Autodesk Inventor part; units mm, degrees
(part 2 of 2)
  spline S29 degree 3 poles (44.5449, -33.6903) (44.3882, -33.8514) (44.153, -34.0929) (43.8555, -34.4298) (43.6383, -34.6876) (43.4284, -34.9513) (43.2262, -35.221) (43.0325, -35.497) (42.8484, -35.7793) (42.6754, -36.0687) (42.5143, -36.3649) (42.3963, -36.6199) (42.3064, -36.8258) (42.2261, -36.9743) (42.1307, -37.1135) (42.0181, -37.2395) (41.9088, -37.3284) (41.8141, -37.3893) (41.7375, -37.4246) (41.6598, -37.4575) (41.5776, -37.4771) (41.4949, -37.4937) (41.4105, -37.496) (41.326, -37.4951) (41.2151, -37.4757) (41.0784, -37.444) (40.9405, -37.4173) (40.8313, -37.39) (40.7538, -37.3564) (40.6776, -37.32) (40.6088, -37.2711) (40.5417, -37.2199) (40.484, -37.1582) (40.4284, -37.0947) (40.3668, -37.0006) (40.303, -36.875) (40.2514, -36.714) (40.2209, -36.548) (40.2079, -36.3798) (40.2096, -36.1551) (40.2054, -35.8742) (40.1788, -35.538) (40.1384, -35.2033) (40.0851, -34.8705) (40.0204, -34.5396) (39.9454, -34.211) (39.8609, -33.8847) (39.7673, -33.5608) (39.6325, -33.1321) (39.5159, -32.8158) (39.4382, -32.6049) knots -1.0784 -1.0784 -1.0784 -1.0784 -1.010995 -0.977291 -0.943586 -0.909882 -0.876178 -0.842474 -0.80877 -0.775067 -0.741365 -0.707665 -0.690816 -0.67397 -0.657123 -0.640284 -0.623449 -0.615023 -0.606598 -0.598176 -0.589749 -0.581327 -0.572901 -0.564477 -0.556053 -0.5392 -0.522347 -0.513923 -0.505499 -0.497074 -0.488651 -0.480225 -0.471802 -0.463377 -0.454951 -0.438116 -0.421277 -0.40443 -0.387584 -0.370735 -0.337035 -0.303333 -0.26963 -0.235926 -0.202222 -0.168518 -0.134814 -0.101109 -0.067405 0 0 0 0 construction
  arc A24 (39.4382, -32.6049) -> (37.971, -32.4507) centre (35.3606, -64.344) ccw construction
  spline S30 degree 3 poles (37.971, -32.4507) (37.8511, -32.6408) (37.6713, -32.9259) (37.4503, -33.3173) (37.2915, -33.6146) (37.141, -33.9162) (36.9993, -34.2221) (36.8672, -34.5323) (36.7458, -34.8467) (36.6368, -35.1657) (36.5408, -35.489) (36.4784, -35.7629) (36.4333, -35.983) (36.3856, -36.1449) (36.3212, -36.3009) (36.2373, -36.4477) (36.1488, -36.5573) (36.0689, -36.6365) (36.0013, -36.687) (35.9321, -36.7354) (35.8558, -36.7716) (35.7783, -36.8051) (35.6962, -36.8249) (35.6135, -36.8416) (35.5009, -36.8456) (35.3606, -36.843) (35.2202, -36.8456) (35.1077, -36.8416) (35.0249, -36.8249) (34.9428, -36.8051) (34.8653, -36.7716) (34.789, -36.7354) (34.7198, -36.687) (34.6523, -36.6365) (34.5723, -36.5573) (34.4839, -36.4477) (34.4, -36.3009) (34.3355, -36.1449) (34.2879, -35.983) (34.2428, -35.7629) (34.1803, -35.489) (34.0844, -35.1657) (33.9753, -34.8467) (33.8539, -34.5323) (33.7219, -34.2221) (33.5802, -33.9162) (33.4297, -33.6146) (33.2709, -33.3173) (33.0498, -32.9259) (32.87, -32.6408) (32.7502, -32.4507) knots -1.0784 -1.0784 -1.0784 -1.0784 -1.010995 -0.977291 -0.943586 -0.909882 -0.876178 -0.842474 -0.80877 -0.775067 -0.741365 -0.707665 -0.690816 -0.67397 -0.657123 -0.640284 -0.623449 -0.615023 -0.606598 -0.598176 -0.589749 -0.581327 -0.572901 -0.564477 -0.556053 -0.5392 -0.522347 -0.513923 -0.505499 -0.497074 -0.488651 -0.480225 -0.471802 -0.463377 -0.454951 -0.438116 -0.421277 -0.40443 -0.387584 -0.370735 -0.337035 -0.303333 -0.26963 -0.235926 -0.202222 -0.168518 -0.134814 -0.101109 -0.067405 0 0 0 0 construction
  arc A25 (32.7502, -32.4507) -> (31.2829, -32.6049) centre (35.3606, -64.344) ccw construction
  spline S31 degree 3 poles (31.2829, -32.6049) (31.2052, -32.8158) (31.0887, -33.1321) (30.9538, -33.5608) (30.8603, -33.8847) (30.7758, -34.211) (30.7008, -34.5396) (30.6361, -34.8705) (30.5827, -35.2033) (30.5424, -35.538) (30.5157, -35.8742) (30.5116, -36.1551) (30.5133, -36.3798) (30.5003, -36.548) (30.4697, -36.714) (30.4181, -36.875) (30.3544, -37.0006) (30.2927, -37.0947) (30.2371, -37.1582) (30.1795, -37.2199) (30.1124, -37.2711) (30.0435, -37.32) (29.9673, -37.3564) (29.8899, -37.39) (29.7806, -37.4173) (29.6428, -37.444) (29.506, -37.4757) (29.3951, -37.4951) (29.3107, -37.496) (29.2263, -37.4937) (29.1435, -37.4771) (29.0614, -37.4575) (28.9836, -37.4246) (28.907, -37.3893) (28.8124, -37.3284) (28.7031, -37.2395) (28.5905, -37.1135) (28.495, -36.9743) (28.4147, -36.8258) (28.3249, -36.6199) (28.2068, -36.3649) (28.0458, -36.0687) (27.8728, -35.7793) (27.6886, -35.497) (27.495, -35.221) (27.2928, -34.9513) (27.0829, -34.6876) (26.8657, -34.4298) (26.5681, -34.0929) (26.333, -33.8514) (26.1762, -33.6903) knots -1.0784 -1.0784 -1.0784 -1.0784 -1.010995 -0.977291 -0.943586 -0.909882 -0.876178 -0.842474 -0.80877 -0.775067 -0.741365 -0.707665 -0.690816 -0.67397 -0.657123 -0.640284 -0.623449 -0.615023 -0.606598 -0.598176 -0.589749 -0.581327 -0.572901 -0.564477 -0.556053 -0.5392 -0.522347 -0.513923 -0.505499 -0.497074 -0.488651 -0.480225 -0.471802 -0.463377 -0.454951 -0.438116 -0.421277 -0.40443 -0.387584 -0.370735 -0.337035 -0.303333 -0.26963 -0.235926 -0.202222 -0.168518 -0.134814 -0.101109 -0.067405 0 0 0 0 construction
  arc A26 (26.1762, -33.6903) -> (24.7731, -34.1463) centre (35.3606, -64.344) ccw construction
  spline S32 degree 3 poles (24.7731, -34.1463) (24.7409, -34.3687) (24.6927, -34.7023) (24.6499, -35.1497) (24.6258, -35.4859) (24.611, -35.8227) (24.6059, -36.1598) (24.6114, -36.4968) (24.6284, -36.8335) (24.6586, -37.1692) (24.7024, -37.5036) (24.7567, -37.7792) (24.8051, -37.9987) (24.8274, -38.1659) (24.832, -38.3347) (24.815, -38.5028) (24.7788, -38.639) (24.738, -38.7439) (24.6968, -38.8175) (24.6533, -38.8898) (24.5983, -38.9539) (24.5411, -39.016) (24.4742, -39.0675) (24.4054, -39.1164) (24.3042, -39.1658) (24.1749, -39.2206) (24.0477, -39.28) (23.9433, -39.3221) (23.8609, -39.3405) (23.7778, -39.3558) (23.6934, -39.3568) (23.609, -39.3548) (23.5261, -39.3387) (23.4438, -39.3201) (23.3386, -39.2802) (23.2132, -39.216) (23.0769, -39.1161) (22.9546, -38.9998) (22.8452, -38.8713) (22.7144, -38.6885) (22.546, -38.4637) (22.3268, -38.2074) (22.0975, -37.9603) (21.8587, -37.7224) (21.6119, -37.4928) (21.358, -37.271) (21.0978, -37.0567) (20.8318, -36.8497) (20.4707, -36.582) (20.1905, -36.3946) (20.0037, -36.2697) knots -1.0784 -1.0784 -1.0784 -1.0784 -1.010995 -0.977291 -0.943586 -0.909882 -0.876178 -0.842474 -0.80877 -0.775067 -0.741365 -0.707665 -0.690816 -0.67397 -0.657123 -0.640284 -0.623449 -0.615023 -0.606598 -0.598176 -0.589749 -0.581327 -0.572901 -0.564477 -0.556053 -0.5392 -0.522347 -0.513923 -0.505499 -0.497074 -0.488651 -0.480225 -0.471802 -0.463377 -0.454951 -0.438116 -0.421277 -0.40443 -0.387584 -0.370735 -0.337035 -0.303333 -0.26963 -0.235926 -0.202222 -0.168518 -0.134814 -0.101109 -0.067405 0 0 0 0 construction
  arc A27 (20.0037, -36.2697) -> (18.726, -37.0074) centre (35.3606, -64.344) ccw construction
  spline S33 degree 3 poles (18.726, -37.0074) (18.7408, -37.2317) (18.7629, -37.568) (18.8141, -38.0146) (18.8604, -38.3484) (18.916, -38.6809) (18.9811, -39.0117) (19.0566, -39.3402) (19.1432, -39.666) (19.2425, -39.9882) (19.3549, -40.3061) (19.4653, -40.5644) (19.5582, -40.769) (19.6148, -40.928) (19.6544, -41.092) (19.6728, -41.2601) (19.6656, -41.4008) (19.6476, -41.5119) (19.6226, -41.5924) (19.595, -41.6722) (19.5546, -41.7463) (19.5115, -41.819) (19.4568, -41.8833) (19.3997, -41.9454) (19.3109, -42.0148) (19.1959, -42.0952) (19.0838, -42.1798) (18.9904, -42.2427) (18.9137, -42.2778) (18.8356, -42.3101) (18.7532, -42.3285) (18.6703, -42.3441) (18.5858, -42.3457) (18.5015, -42.3445) (18.3903, -42.3274) (18.2542, -42.2907) (18.1001, -42.2213) (17.9563, -42.133) (17.8226, -42.03) (17.6567, -41.8784) (17.4452, -41.6935) (17.1775, -41.4884) (16.9018, -41.2944) (16.6188, -41.1114) (16.3296, -40.9381) (16.0352, -40.7739) (15.7361, -40.6184) (15.4329, -40.4712) (15.0241, -40.2845) (14.711, -40.1594) (14.5023, -40.0761) knots -1.0784 -1.0784 -1.0784 -1.0784 -1.010995 -0.977291 -0.943586 -0.909882 -0.876178 -0.842474 -0.80877 -0.775067 -0.741365 -0.707665 -0.690816 -0.67397 -0.657123 -0.640284 -0.623449 -0.615023 -0.606598 -0.598176 -0.589749 -0.581327 -0.572901 -0.564477 -0.556053 -0.5392 -0.522347 -0.513923 -0.505499 -0.497074 -0.488651 -0.480225 -0.471802 -0.463377 -0.454951 -0.438116 -0.421277 -0.40443 -0.387584 -0.370735 -0.337035 -0.303333 -0.26963 -0.235926 -0.202222 -0.168518 -0.134814 -0.101109 -0.067405 0 0 0 0 construction
  arc A28 (14.5023, -40.0761) -> (13.4059, -41.0633) centre (35.3606, -64.344) ccw construction
  spline S34 degree 3 poles (13.4059, -41.0633) (13.467, -41.2796) (13.5586, -41.604) (13.7015, -42.0301) (13.8162, -42.3471) (13.9397, -42.6608) (14.0721, -42.9707) (14.2143, -43.2764) (14.3667, -43.5771) (14.5308, -43.8715) (14.7069, -44.1591) (14.8686, -44.3888) (15.002, -44.5696) (15.0904, -44.7134) (15.1633, -44.8657) (15.2162, -45.0262) (15.2385, -45.1653) (15.2439, -45.2777) (15.2362, -45.3617) (15.2258, -45.4455) (15.2016, -45.5264) (15.1747, -45.6064) (15.1344, -45.6807) (15.0915, -45.7533) (15.0192, -45.8397) (14.9233, -45.9422) (14.8313, -46.0483) (14.753, -46.1292) (14.6853, -46.1795) (14.6156, -46.2273) (14.5389, -46.2625) (14.4609, -46.295) (14.3787, -46.314) (14.2959, -46.3305) (14.1836, -46.3368) (14.0429, -46.3292) (13.8777, -46.2934) (13.7187, -46.2369) (13.5665, -46.164) (13.3727, -46.0502) (13.1274, -45.9133) (12.8229, -45.7683) (12.5129, -45.6359) (12.198, -45.5157) (11.8791, -45.4063) (11.557, -45.307) (11.2321, -45.217) (10.9049, -45.1361) (10.4662, -45.0384) (10.134, -44.9812) (9.9125, -44.9431) knots -1.0784 -1.0784 -1.0784 -1.0784 -1.010995 -0.977291 -0.943586 -0.909882 -0.876178 -0.842474 -0.80877 -0.775067 -0.741365 -0.707665 -0.690816 -0.67397 -0.657123 -0.640284 -0.623449 -0.615023 -0.606598 -0.598176 -0.589749 -0.581327 -0.572901 -0.564477 -0.556053 -0.5392 -0.522347 -0.513923 -0.505499 -0.497074 -0.488651 -0.480225 -0.471802 -0.463377 -0.454951 -0.438116 -0.421277 -0.40443 -0.387584 -0.370735 -0.337035 -0.303333 -0.26963 -0.235926 -0.202222 -0.168518 -0.134814 -0.101109 -0.067405 0 0 0 0 construction
  arc A29 (9.9125, -44.9431) -> (9.0453, -46.1367) centre (35.3606, -64.344) ccw construction
  spline S35 degree 3 poles (9.0453, -46.1367) (9.15, -46.3355) (9.3071, -46.6338) (9.5355, -47.0209) (9.7136, -47.3071) (9.8996, -47.5882) (10.0936, -47.8639) (10.2962, -48.1333) (10.5078, -48.3957) (10.7295, -48.6497) (10.9615, -48.8944) (11.1675, -49.0854) (11.3356, -49.2345) (11.452, -49.3568) (11.5549, -49.4906) (11.64, -49.6366) (11.6907, -49.768) (11.7194, -49.8769) (11.7293, -49.9606) (11.7366, -50.0447) (11.7298, -50.1289) (11.72, -50.2128) (11.6961, -50.2938) (11.6692, -50.3738) (11.6164, -50.4732) (11.544, -50.5935) (11.476, -50.7163) (11.4163, -50.8118) (11.3605, -50.8751) (11.3023, -50.9363) (11.2345, -50.9867) (11.165, -51.0347) (11.0885, -51.0704) (11.011, -51.1037) (10.9025, -51.1333) (10.7633, -51.1551) (10.5942, -51.1544) (10.4269, -51.1322) (10.2629, -51.0925) (10.0497, -51.0215) (9.7813, -50.9386) (9.4533, -50.8601) (9.1226, -50.795) (8.7895, -50.7429) (8.4549, -50.7022) (8.1191, -50.672) (7.7827, -50.6515) (7.4458, -50.6404) (6.9963, -50.6361) (6.6595, -50.6493) (6.4349, -50.658) knots -1.0784 -1.0784 -1.0784 -1.0784 -1.010995 -0.977291 -0.943586 -0.909882 -0.876178 -0.842474 -0.80877 -0.775067 -0.741365 -0.707665 -0.690816 -0.67397 -0.657123 -0.640284 -0.623449 -0.615023 -0.606598 -0.598176 -0.589749 -0.581327 -0.572901 -0.564477 -0.556053 -0.5392 -0.522347 -0.513923 -0.505499 -0.497074 -0.488651 -0.480225 -0.471802 -0.463377 -0.454951 -0.438116 -0.421277 -0.40443 -0.387584 -0.370735 -0.337035 -0.303333 -0.26963 -0.235926 -0.202222 -0.168518 -0.134814 -0.101109 -0.067405 0 0 0 0 construction
  arc A30 (6.4349, -50.658) -> (5.8348, -52.0058) centre (35.3606, -64.344) ccw construction
  spline S36 degree 3 poles (5.8348, -52.0058) (5.9786, -52.1785) (6.1943, -52.4376) (6.4982, -52.7688) (6.7319, -53.0117) (6.9722, -53.248) (7.2193, -53.4773) (7.4735, -53.6988) (7.7351, -53.9114) (8.0047, -54.1137) (8.2825, -54.3048) (8.5237, -54.4489) (8.7192, -54.5598) (8.8584, -54.6552) (8.9869, -54.7646) (9.1005, -54.8898) (9.1774, -55.0078) (9.2281, -55.1083) (9.2552, -55.1881) (9.2798, -55.2689) (9.2907, -55.3526) (9.2986, -55.4367) (9.292, -55.5209) (9.2823, -55.6048) (9.2514, -55.713) (9.2055, -55.8457) (9.1646, -55.98) (9.126, -56.0858) (9.0846, -56.1594) (9.0404, -56.2313) (8.9846, -56.2947) (8.9266, -56.3561) (8.8592, -56.4069) (8.7903, -56.4556) (8.6903, -56.5071) (8.5587, -56.5574) (8.3932, -56.5918) (8.2249, -56.6049) (8.0562, -56.6002) (7.8329, -56.5751) (7.5531, -56.5498) (7.216, -56.5412) (6.8789, -56.5463) (6.5423, -56.5646) (6.2065, -56.5943) (5.8719, -56.6346) (5.5385, -56.6845) (5.2067, -56.7437) (4.7661, -56.833) (4.4394, -56.9158) (4.2215, -56.971) knots -1.0784 -1.0784 -1.0784 -1.0784 -1.010995 -0.977291 -0.943586 -0.909882 -0.876178 -0.842474 -0.80877 -0.775067 -0.741365 -0.707665 -0.690816 -0.67397 -0.657123 -0.640284 -0.623449 -0.615023 -0.606598 -0.598176 -0.589749 -0.581327 -0.572901 -0.564477 -0.556053 -0.5392 -0.522347 -0.513923 -0.505499 -0.497074 -0.488651 -0.480225 -0.471802 -0.463377 -0.454951 -0.438116 -0.421277 -0.40443 -0.387584 -0.370735 -0.337035 -0.303333 -0.26963 -0.235926 -0.202222 -0.168518 -0.134814 -0.101109 -0.067405 0 0 0 0 construction
  arc A31 (4.2215, -56.971) -> (3.9148, -58.4142) centre (35.3606, -64.344) ccw construction
  spline S37 degree 3 poles (3.9148, -58.4142) (4.0913, -58.5532) (4.3561, -58.7618) (4.7223, -59.0226) (5.0013, -59.2116) (5.2856, -59.3928) (5.575, -59.5657) (5.8696, -59.7294) (6.1697, -59.8831) (6.4755, -60.0249) (6.787, -60.1541) (7.0529, -60.2448) (7.2671, -60.3127) (7.4231, -60.377) (7.5715, -60.4574) (7.7087, -60.5562) (7.8085, -60.6556) (7.8789, -60.7434) (7.9221, -60.8158) (7.9629, -60.8897) (7.9909, -60.9694) (8.0161, -61.05) (8.0272, -61.1337) (8.0352, -61.2177) (8.0274, -61.3301) (8.0102, -61.4694) (7.9981, -61.6092) (7.9824, -61.7208) (7.9571, -61.8013) (7.9288, -61.8809) (7.8874, -61.9545) (7.8435, -62.0265) (7.7881, -62.0903) (7.7308, -62.1522) (7.6437, -62.2234) (7.5254, -62.2999) (7.3707, -62.3681) (7.2088, -62.4158) (7.0428, -62.4463) (6.8192, -62.4681) (6.5403, -62.5016) (6.2087, -62.5633) (5.8801, -62.6384) (5.5546, -62.7262) (5.2324, -62.8251) (4.9134, -62.9341) (4.5977, -63.0523) (4.2854, -63.1791) (3.8731, -63.358) (3.5707, -63.507) (3.3691, -63.6063) knots -1.0784 -1.0784 -1.0784 -1.0784 -1.010995 -0.977291 -0.943586 -0.909882 -0.876178 -0.842474 -0.80877 -0.775067 -0.741365 -0.707665 -0.690816 -0.67397 -0.657123 -0.640284 -0.623449 -0.615023 -0.606598 -0.598176 -0.589749 -0.581327 -0.572901 -0.564477 -0.556053 -0.5392 -0.522347 -0.513923 -0.505499 -0.497074 -0.488651 -0.480225 -0.471802 -0.463377 -0.454951 -0.438116 -0.421277 -0.40443 -0.387584 -0.370735 -0.337035 -0.303333 -0.26963 -0.235926 -0.202222 -0.168518 -0.134814 -0.101109 -0.067405 0 0 0 0 construction
  arc A32 (3.3691, -63.6063) -> (3.3691, -65.0817) centre (35.3606, -64.344) ccw construction
  spline S38 degree 3 poles (3.3691, -65.0817) (3.5707, -65.181) (3.8731, -65.33) (4.2854, -65.5089) (4.5977, -65.6358) (4.9134, -65.7539) (5.2324, -65.8629) (5.5546, -65.9618) (5.8801, -66.0497) (6.2087, -66.1248) (6.5403, -66.1864) (6.8192, -66.2199) (7.0428, -66.2417) (7.2088, -66.2722) (7.3707, -66.32) (7.5254, -66.3881) (7.6437, -66.4646) (7.7308, -66.5358) (7.7881, -66.5977) (7.8435, -66.6615) (7.8874, -66.7336) (7.9288, -66.8072) (7.9571, -66.8867) (7.9824, -66.9673) (7.9981, -67.0788) (8.0102, -67.2187) (8.0274, -67.358) (8.0352, -67.4703) (8.0272, -67.5544) (8.0161, -67.6381) (7.9909, -67.7187) (7.9629, -67.7983) (7.9221, -67.8722) (7.8789, -67.9447) (7.8085, -68.0324) (7.7087, -68.1319) (7.5715, -68.2307) (7.4231, -68.311) (7.2671, -68.3754) (7.0529, -68.4432) (6.787, -68.534) (6.4755, -68.6632) (6.1697, -68.805) (5.8696, -68.9586) (5.575, -69.1223) (5.2856, -69.2952) (5.0013, -69.4764) (4.7223, -69.6655) (4.3561, -69.9262) (4.0913, -70.1348) (3.9148, -70.2739) knots -1.0784 -1.0784 -1.0784 -1.0784 -1.010995 -0.977291 -0.943586 -0.909882 -0.876178 -0.842474 -0.80877 -0.775067 -0.741365 -0.707665 -0.690816 -0.67397 -0.657123 -0.640284 -0.623449 -0.615023 -0.606598 -0.598176 -0.589749 -0.581327 -0.572901 -0.564477 -0.556053 -0.5392 -0.522347 -0.513923 -0.505499 -0.497074 -0.488651 -0.480225 -0.471802 -0.463377 -0.454951 -0.438116 -0.421277 -0.40443 -0.387584 -0.370735 -0.337035 -0.303333 -0.26963 -0.235926 -0.202222 -0.168518 -0.134814 -0.101109 -0.067405 0 0 0 0 construction
  arc A33 (3.9148, -70.2739) -> (4.2215, -71.717) centre (35.3606, -64.344) ccw construction
  spline S39 degree 3 poles (4.2215, -71.717) (4.4394, -71.7722) (4.7661, -71.8551) (5.2067, -71.9444) (5.5385, -72.0035) (5.8719, -72.0534) (6.2065, -72.0937) (6.5423, -72.1235) (6.8789, -72.1417) (7.216, -72.1469) (7.5531, -72.1382) (7.8329, -72.113) (8.0562, -72.0879) (8.2249, -72.0832) (8.3932, -72.0962) (8.5587, -72.1307) (8.6903, -72.1809) (8.7903, -72.2324) (8.8592, -72.2811) (8.9266, -72.332) (8.9846, -72.3934) (9.0404, -72.4567) (9.0846, -72.5287) (9.126, -72.6022) (9.1646, -72.708) (9.2055, -72.8423) (9.2514, -72.975) (9.2823, -73.0833) (9.292, -73.1671) (9.2986, -73.2513) (9.2907, -73.3354) (9.2798, -73.4191) (9.2552, -73.4999) (9.2281, -73.5798) (9.1774, -73.6802) (9.1005, -73.7983) (8.9869, -73.9234) (8.8584, -74.0329) (8.7192, -74.1282) (8.5237, -74.2392) (8.2825, -74.3832) (8.0047, -74.5743) (7.7351, -74.7766) (7.4735, -74.9893) (7.2193, -75.2107) (6.9722, -75.44) (6.7319, -75.6763) (6.4982, -75.9192) (6.1943, -76.2504) (5.9786, -76.5095) (5.8348, -76.6822) knots -1.0784 -1.0784 -1.0784 -1.0784 -1.010995 -0.977291 -0.943586 -0.909882 -0.876178 -0.842474 -0.80877 -0.775067 -0.741365 -0.707665 -0.690816 -0.67397 -0.657123 -0.640284 -0.623449 -0.615023 -0.606598 -0.598176 -0.589749 -0.581327 -0.572901 -0.564477 -0.556053 -0.5392 -0.522347 -0.513923 -0.505499 -0.497074 -0.488651 -0.480225 -0.471802 -0.463377 -0.454951 -0.438116 -0.421277 -0.40443 -0.387584 -0.370735 -0.337035 -0.303333 -0.26963 -0.235926 -0.202222 -0.168518 -0.134814 -0.101109 -0.067405 0 0 0 0 construction
  arc A34 (5.8348, -76.6822) -> (6.4349, -78.03) centre (35.3606, -64.344) ccw construction
  spline S40 degree 3 poles (6.4349, -78.03) (6.6595, -78.0388) (6.9963, -78.0519) (7.4458, -78.0476) (7.7827, -78.0365) (8.1191, -78.016) (8.4549, -77.9858) (8.7895, -77.9451) (9.1226, -77.893) (9.4533, -77.828) (9.7813, -77.7494) (10.0497, -77.6665) (10.2629, -77.5955) (10.4269, -77.5559) (10.5942, -77.5336) (10.7633, -77.533) (10.9025, -77.5547) (11.011, -77.5843) (11.0885, -77.6176) (11.165, -77.6534) (11.2345, -77.7013) (11.3023, -77.7517) (11.3605, -77.8129) (11.4163, -77.8762) (11.476, -77.9717) (11.544, -78.0945) (11.6164, -78.2148) (11.6692, -78.3143) (11.6961, -78.3943) (11.72, -78.4753) (11.7298, -78.5592) (11.7366, -78.6433) (11.7293, -78.7274) (11.7194, -78.8112) (11.6907, -78.92) (11.64, -79.0514) (11.5549, -79.1975) (11.452, -79.3313) (11.3356, -79.4535) (11.1675, -79.6026) (10.9615, -79.7937) (10.7295, -80.0384) (10.5078, -80.2923) (10.2962, -80.5547) (10.0936, -80.8241) (9.8996, -81.0998) (9.7136, -81.3809) (9.5355, -81.6671) (9.3071, -82.0542) (9.15, -82.3525) (9.0453, -82.5513) knots -1.0784 -1.0784 -1.0784 -1.0784 -1.010995 -0.977291 -0.943586 -0.909882 -0.876178 -0.842474 -0.80877 -0.775067 -0.741365 -0.707665 -0.690816 -0.67397 -0.657123 -0.640284 -0.623449 -0.615023 -0.606598 -0.598176 -0.589749 -0.581327 -0.572901 -0.564477 -0.556053 -0.5392 -0.522347 -0.513923 -0.505499 -0.497074 -0.488651 -0.480225 -0.471802 -0.463377 -0.454951 -0.438116 -0.421277 -0.40443 -0.387584 -0.370735 -0.337035 -0.303333 -0.26963 -0.235926 -0.202222 -0.168518 -0.134814 -0.101109 -0.067405 0 0 0 0 construction
  arc A35 (9.0453, -82.5513) -> (9.9125, -83.7449) centre (35.3606, -64.344) ccw construction
  spline S41 degree 3 poles (9.9125, -83.7449) (10.134, -83.7068) (10.4662, -83.6496) (10.9049, -83.552) (11.2321, -83.4711) (11.557, -83.3811) (11.8791, -83.2817) (12.198, -83.1723) (12.5129, -83.0521) (12.8229, -82.9197) (13.1274, -82.7747) (13.3727, -82.6378) (13.5665, -82.5241) (13.7187, -82.4511) (13.8777, -82.3946) (14.0429, -82.3588) (14.1836, -82.3512) (14.2959, -82.3576) (14.3787, -82.374) (14.4609, -82.3931) (14.5389, -82.4255) (14.6156, -82.4607) (14.6853, -82.5085) (14.753, -82.5588) (14.8313, -82.6398) (14.9233, -82.7458) (15.0192, -82.8484) (15.0915, -82.9347) (15.1344, -83.0074) (15.1747, -83.0816) (15.2016, -83.1616) (15.2258, -83.2425) (15.2362, -83.3263) (15.2439, -83.4103) (15.2385, -83.5227) (15.2162, -83.6618) (15.1633, -83.8224) (15.0904, -83.9746) (15.002, -84.1184) (14.8686, -84.2992) (14.7069, -84.5289) (14.5308, -84.8165) (14.3667, -85.111) (14.2143, -85.4116) (14.0721, -85.7173) (13.9397, -86.0273) (13.8162, -86.341) (13.7015, -86.6579) (13.5586, -87.084) (13.467, -87.4085) (13.4059, -87.6247) knots -1.0784 -1.0784 -1.0784 -1.0784 -1.010995 -0.977291 -0.943586 -0.909882 -0.876178 -0.842474 -0.80877 -0.775067 -0.741365 -0.707665 -0.690816 -0.67397 -0.657123 -0.640284 -0.623449 -0.615023 -0.606598 -0.598176 -0.589749 -0.581327 -0.572901 -0.564477 -0.556053 -0.5392 -0.522347 -0.513923 -0.505499 -0.497074 -0.488651 -0.480225 -0.471802 -0.463377 -0.454951 -0.438116 -0.421277 -0.40443 -0.387584 -0.370735 -0.337035 -0.303333 -0.26963 -0.235926 -0.202222 -0.168518 -0.134814 -0.101109 -0.067405 0 0 0 0 construction
  arc A36 (13.4059, -87.6247) -> (14.5023, -88.6119) centre (35.3606, -64.344) ccw construction
  spline S42 degree 3 poles (14.5023, -88.6119) (14.711, -88.5286) (15.0241, -88.4036) (15.4329, -88.2169) (15.7361, -88.0697) (16.0352, -87.9141) (16.3296, -87.75) (16.6188, -87.5767) (16.9018, -87.3936) (17.1775, -87.1996) (17.4452, -86.9945) (17.6567, -86.8096) (17.8226, -86.658) (17.9563, -86.5551) (18.1001, -86.4667) (18.2542, -86.3973) (18.3903, -86.3606) (18.5015, -86.3435) (18.5858, -86.3424) (18.6703, -86.3439) (18.7532, -86.3595) (18.8356, -86.378) (18.9137, -86.4102) (18.9904, -86.4453) (19.0838, -86.5082) (19.1959, -86.5928) (19.3109, -86.6732) (19.3997, -86.7426) (19.4568, -86.8048) (19.5115, -86.8691) (19.5546, -86.9417) (19.595, -87.0158) (19.6226, -87.0956) (19.6476, -87.1762) (19.6656, -87.2873) (19.6728, -87.428) (19.6544, -87.596) (19.6148, -87.7601) (19.5582, -87.9191) (19.4653, -88.1236) (19.3549, -88.382) (19.2425, -88.6999) (19.1432, -89.022) (19.0566, -89.3478) (18.9811, -89.6764) (18.916, -90.0071) (18.8604, -90.3396) (18.8141, -90.6735) (18.7629, -91.12) (18.7408, -91.4564) (18.726, -91.6806) knots -1.0784 -1.0784 -1.0784 -1.0784 -1.010995 -0.977291 -0.943586 -0.909882 -0.876178 -0.842474 -0.80877 -0.775067 -0.741365 -0.707665 -0.690816 -0.67397 -0.657123 -0.640284 -0.623449 -0.615023 -0.606598 -0.598176 -0.589749 -0.581327 -0.572901 -0.564477 -0.556053 -0.5392 -0.522347 -0.513923 -0.505499 -0.497074 -0.488651 -0.480225 -0.471802 -0.463377 -0.454951 -0.438116 -0.421277 -0.40443 -0.387584 -0.370735 -0.337035 -0.303333 -0.26963 -0.235926 -0.202222 -0.168518 -0.134814 -0.101109 -0.067405 0 0 0 0 construction
  arc A37 (18.726, -91.6806) -> (20.0037, -92.4183) centre (35.3606, -64.344) ccw construction
  spline S43 degree 3 poles (20.0037, -92.4183) (20.1905, -92.2934) (20.4707, -92.106) (20.8318, -91.8384) (21.0978, -91.6314) (21.358, -91.417) (21.6119, -91.1953) (21.8587, -90.9656) (22.0975, -90.7277) (22.3268, -90.4806) (22.546, -90.2243) (22.7144, -89.9995) (22.8452, -89.8168) (22.9546, -89.6883) (23.0769, -89.5719) (23.2132, -89.472) (23.3386, -89.4078) (23.4438, -89.368) (23.5261, -89.3493) (23.609, -89.3333) (23.6934, -89.3313) (23.7778, -89.3322) (23.8609, -89.3475) (23.9433, -89.3659) (24.0477, -89.408) (24.1749, -89.4675) (24.3042, -89.5222) (24.4054, -89.5716) (24.4742, -89.6205) (24.5411, -89.672) (24.5983, -89.7342) (24.6533, -89.7982) (24.6968, -89.8706) (24.738, -89.9442) (24.7788, -90.0491) (24.815, -90.1852) (24.832, -90.3534) (24.8274, -90.5221) (24.8051, -90.6894) (24.7567, -90.9088) (24.7024, -91.1844) (24.6586, -91.5188) (24.6284, -91.8545) (24.6114, -92.1912) (24.6059, -92.5283) (24.611, -92.8653) (24.6258, -93.2021) (24.6499, -93.5383) (24.6927, -93.9857) (24.7409, -94.3194) (24.7731, -94.5418) knots -1.0784 -1.0784 -1.0784 -1.0784 -1.010995 -0.977291 -0.943586 -0.909882 -0.876178 -0.842474 -0.80877 -0.775067 -0.741365 -0.707665 -0.690816 -0.67397 -0.657123 -0.640284 -0.623449 -0.615023 -0.606598 -0.598176 -0.589749 -0.581327 -0.572901 -0.564477 -0.556053 -0.5392 -0.522347 -0.513923 -0.505499 -0.497074 -0.488651 -0.480225 -0.471802 -0.463377 -0.454951 -0.438116 -0.421277 -0.40443 -0.387584 -0.370735 -0.337035 -0.303333 -0.26963 -0.235926 -0.202222 -0.168518 -0.134814 -0.101109 -0.067405 0 0 0 0 construction
  arc A38 (24.7731, -94.5418) -> (26.1762, -94.9977) centre (35.3606, -64.344) ccw construction
  spline S44 degree 3 poles (26.1762, -94.9977) (26.333, -94.8367) (26.5681, -94.5951) (26.8657, -94.2583) (27.0829, -94.0005) (27.2928, -93.7367) (27.495, -93.467) (27.6886, -93.1911) (27.8728, -92.9087) (28.0458, -92.6194) (28.2068, -92.3231) (28.3249, -92.0682) (28.4147, -91.8622) (28.495, -91.7138) (28.5905, -91.5746) (28.7031, -91.4485) (28.8124, -91.3596) (28.907, -91.2988) (28.9836, -91.2634) (29.0614, -91.2305) (29.1435, -91.211) (29.2263, -91.1943) (29.3107, -91.192) (29.3951, -91.1929) (29.506, -91.2124) (29.6428, -91.2441) (29.7806, -91.2707) (29.8899, -91.2981) (29.9673, -91.3316) (30.0435, -91.368) (30.1124, -91.4169) (30.1795, -91.4681) (30.2371, -91.5299) (30.2927, -91.5933) (30.3544, -91.6874) (30.4181, -91.813) (30.4697, -91.974) (30.5003, -92.14) (30.5133, -92.3083) (30.5116, -92.533) (30.5157, -92.8139) (30.5424, -93.15) (30.5827, -93.4847) (30.6361, -93.8176) (30.7008, -94.1484) (30.7758, -94.477) (30.8603, -94.8034) (30.9538, -95.1272) (31.0887, -95.556) (31.2052, -95.8723) (31.2829, -96.0832) knots -1.0784 -1.0784 -1.0784 -1.0784 -1.010995 -0.977291 -0.943586 -0.909882 -0.876178 -0.842474 -0.80877 -0.775067 -0.741365 -0.707665 -0.690816 -0.67397 -0.657123 -0.640284 -0.623449 -0.615023 -0.606598 -0.598176 -0.589749 -0.581327 -0.572901 -0.564477 -0.556053 -0.5392 -0.522347 -0.513923 -0.505499 -0.497074 -0.488651 -0.480225 -0.471802 -0.463377 -0.454951 -0.438116 -0.421277 -0.40443 -0.387584 -0.370735 -0.337035 -0.303333 -0.26963 -0.235926 -0.202222 -0.168518 -0.134814 -0.101109 -0.067405 0 0 0 0 construction
  arc A39 (31.2829, -96.0832) -> (32.7502, -96.2374) centre (35.3606, -64.344) ccw construction
  spline S45 degree 3 poles (32.7502, -96.2374) (32.87, -96.0473) (33.0498, -95.7621) (33.2709, -95.3707) (33.4297, -95.0734) (33.5802, -94.7718) (33.7219, -94.4659) (33.8539, -94.1558) (33.9753, -93.8413) (34.0844, -93.5223) (34.1803, -93.199) (34.2428, -92.9251) (34.2879, -92.705) (34.3355, -92.5431) (34.4, -92.3871) (34.4839, -92.2404) (34.5723, -92.1307) (34.6523, -92.0515) (34.7198, -92.001) (34.789, -91.9526) (34.8653, -91.9165) (34.9428, -91.883) (35.0249, -91.8632) (35.1077, -91.8465) (35.2202, -91.8425) (35.3606, -91.845) (35.5009, -91.8425) (35.6135, -91.8465) (35.6962, -91.8632) (35.7783, -91.883) (35.8558, -91.9165) (35.9321, -91.9526) (36.0013, -92.001) (36.0689, -92.0515) (36.1488, -92.1307) (36.2373, -92.2404) (36.3212, -92.3871) (36.3856, -92.5431) (36.4333, -92.705) (36.4784, -92.9251) (36.5408, -93.199) (36.6368, -93.5223) (36.7458, -93.8413) (36.8672, -94.1558) (36.9993, -94.4659) (37.141, -94.7718) (37.2915, -95.0734) (37.4503, -95.3707) (37.6713, -95.7621) (37.8511, -96.0473) (37.971, -96.2374) knots -1.0784 -1.0784 -1.0784 -1.0784 -1.010995 -0.977291 -0.943586 -0.909882 -0.876178 -0.842474 -0.80877 -0.775067 -0.741365 -0.707665 -0.690816 -0.67397 -0.657123 -0.640284 -0.623449 -0.615023 -0.606598 -0.598176 -0.589749 -0.581327 -0.572901 -0.564477 -0.556053 -0.5392 -0.522347 -0.513923 -0.505499 -0.497074 -0.488651 -0.480225 -0.471802 -0.463377 -0.454951 -0.438116 -0.421277 -0.40443 -0.387584 -0.370735 -0.337035 -0.303333 -0.26963 -0.235926 -0.202222 -0.168518 -0.134814 -0.101109 -0.067405 0 0 0 0 construction
  arc A40 (37.971, -96.2374) -> (39.4382, -96.0832) centre (35.3606, -64.344) ccw construction
  circle A41 centre (35.3606, -64.344) radius 5.767 construction
  circle A42 centre (35.3606, -64.344) radius 4.14 construction
  line L37 (58.171, -15.7835) -> (-0.0002, -15.7835)
  line L38 (-0.0002, -15.7835) -> (-0.0002, -123.1057)
  line L39 (-0.0002, -123.1057) -> (58.171, -123.1057)
  line L40 (58.171, -123.1057) -> (58.171, -15.7835)
  line L41 (58.171, -25.7835) -> (-0.0002, -25.7835)
  dimension "d8" = 1
  dimension "d21" = 10
  constraints: 10 end point, 4 point on line, 2 parallel, 2 perpendicular, 1 horizontal
  measures "d8" distance between parallel lines of L24 L41
  measures "d21" distance between parallel lines of L37 L41
extrude "Extrusion1" add sketch "Sketch1" along normal blind 5 and the other way blind 9.75
sketch "Sketch5" plane through (-0.0002, -123.1057, 5) normal (0, -1, 0) x (1, 0, 0)
  line L0 (58.1712, -5.729) -> (56.0979, -5.729) projected
  arc A0 (56.0979, -5.729) -> (48.1592, -5.0001) centre (47.5772, -54.9369) ccw projected
  line L1 (48.1592, -5.0001) -> (48.1592, -5.9194) projected
  line L2 (48.1592, -5.9194) -> (46.2813, -5.9194) projected
  arc A1 (46.2813, -5.9194) -> (40.6924, -5.4904) centre (41.5081, -31.4831) ccw projected
  arc A2 (40.6924, -5.4904) -> (32.7872, -6.7551) centre (40.2264, -27.9175) ccw projected
  arc A3 (22.1478, -6.9292) -> (32.7872, -6.7551) centre (27.1272, 13.9496) ccw projected
  line L3 (22.1478, -6.9292) -> (20.1773, -6.9292) projected
  line L4 (20.1773, -6.9292) -> (20.1773, -8.0939) projected
  line L5 (20.1773, -8.0939) -> (16.4523, -8.0939) projected
  arc A4 (16.4523, -8.0939) -> (8.2145, -7.8887) centre (11.783, -30.0814) ccw projected
  arc A5 (6.4215, -7.7683) -> (8.2145, -7.8887) centre (7.6247, -3.2574) ccw projected
  line L6 (6.4215, -7.7683) -> (6.4215, -7.4041) projected
  arc A6 (6.4215, -7.4041) -> (1.9312, -7.8628) centre (9.2045, -56.8579) ccw projected
  line L7 (1.9312, -7.8628) -> (0, -7.7332) projected
  line L8 (0, -7.7332) -> (0, -14.8132) projected
  line L9 (0, -14.8132) -> (-6.11, -14.8132) projected
  line L10 (-6.11, -14.8132) -> (-6.11, -23.749) projected
  line L11 (-6.11, -23.749) -> (58.1712, -23.749) projected
  line L12 (58.1712, -23.749) -> (58.1712, -5.729) projected
  point P0 (58.1712, 0)
extrude "Extrusion5" cut sketch "Sketch5" against normal blind 202.5
sketch "Sketch6" plane through (0, 0, 5) normal (0, 0, 1) x (1, 0, 0)
  circle A0 centre (53.171, -20.7837) radius 1.25 projected
  circle A1 centre (5, -20.7837) radius 1.25 projected
  circle A2 centre (53.171, -118.1057) radius 1.25 projected
  circle A3 centre (5, -118.1057) radius 1.25 projected
  point P0 (0, 0)
extrude "Extrusion6" cut sketch "Sketch6" against normal blind 4
body "Solid1"
